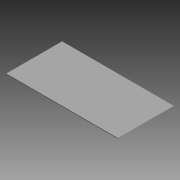
# Autodesk Inventor part: Abtropfgitter
Saved by Autodesk Inventor 2013 (Build 170138000, 138)
## iProperties
Created: 2012-07-26
Part Number: Abtropfgitter
Material: Allgemein
Document SubType Name: Modeling
Designer: fivef
Density: 1 g/cm^3
Mass: 14.3451 g
Surface Area: 368.301 cm^2
Volume: 14.3451 cm^3
Author: fivef
Autodesk Inventor part; units mm, degrees
ref_plane "YZ Plane" through (0, 0, 0) normal (1, 0, 0) x (0, 1, 0)
ref_plane "XZ Plane" through (0, 0, 0) normal (0, 1, 0) x (-1, 0, 0)
ref_plane "XY Plane" through (0, 0, 0) normal (0, 0, 1) x (1, 0, 0)
sketch "Skizze2" plane through (0, 0, 0) normal (0, 0, 1) x (1, 0, 0)
  line L0 (-100, 50) -> (100, 50)
  line L1 (100, 50) -> (100, -50)
  line L2 (100, -50) -> (-100, -50)
  line L3 (-100, -50) -> (-100, 50)
  line L4 (-100, 50) -> (100, -50) construction
  line L5 (100, 50) -> (-100, -50) construction
  circle A0 centre (-98, 48) radius 1.5
  circle A1 centre (-93, 48) radius 1.5
  circle A2 centre (-88, 48) radius 1.5
  circle A3 centre (-83, 48) radius 1.5
  circle A4 centre (-78, 48) radius 1.5
  circle A5 centre (-73, 48) radius 1.5
  circle A6 centre (-68, 48) radius 1.5
  circle A7 centre (-63, 48) radius 1.5
  circle A8 centre (-58, 48) radius 1.5
  circle A9 centre (-53, 48) radius 1.5
  circle A10 centre (-48, 48) radius 1.5
  circle A11 centre (-43, 48) radius 1.5
  circle A12 centre (-38, 48) radius 1.5
  circle A13 centre (-33, 48) radius 1.5
  circle A14 centre (-28, 48) radius 1.5
  circle A15 centre (-23, 48) radius 1.5
  circle A16 centre (-18, 48) radius 1.5
  circle A17 centre (-13, 48) radius 1.5
  circle A18 centre (-8, 48) radius 1.5
  circle A19 centre (-3, 48) radius 1.5
  circle A20 centre (2, 48) radius 1.5
  circle A21 centre (7, 48) radius 1.5
  circle A22 centre (12, 48) radius 1.5
  circle A23 centre (17, 48) radius 1.5
  circle A24 centre (22, 48) radius 1.5
  circle A25 centre (27, 48) radius 1.5
  circle A26 centre (32, 48) radius 1.5
  circle A27 centre (37, 48) radius 1.5
  circle A28 centre (42, 48) radius 1.5
  circle A29 centre (47, 48) radius 1.5
  circle A30 centre (52, 48) radius 1.5
  circle A31 centre (57, 48) radius 1.5
  circle A32 centre (62, 48) radius 1.5
  circle A33 centre (67, 48) radius 1.5
  circle A34 centre (72, 48) radius 1.5
  circle A35 centre (77, 48) radius 1.5
  circle A36 centre (82, 48) radius 1.5
  circle A37 centre (87, 48) radius 1.5
  circle A38 centre (92, 48) radius 1.5
  circle A39 centre (97, 48) radius 1.5
  circle A40 centre (-98, 43) radius 1.5
  circle A41 centre (-93, 43) radius 1.5
  circle A42 centre (-88, 43) radius 1.5
  circle A43 centre (-83, 43) radius 1.5
  circle A44 centre (-78, 43) radius 1.5
  circle A45 centre (-73, 43) radius 1.5
  circle A46 centre (-68, 43) radius 1.5
  circle A47 centre (-63, 43) radius 1.5
  circle A48 centre (-58, 43) radius 1.5
  circle A49 centre (-53, 43) radius 1.5
  circle A50 centre (-48, 43) radius 1.5
  circle A51 centre (-43, 43) radius 1.5
  circle A52 centre (-38, 43) radius 1.5
  circle A53 centre (-33, 43) radius 1.5
  circle A54 centre (-28, 43) radius 1.5
  circle A55 centre (-23, 43) radius 1.5
  circle A56 centre (-18, 43) radius 1.5
  circle A57 centre (-13, 43) radius 1.5
  circle A58 centre (-8, 43) radius 1.5
  circle A59 centre (-3, 43) radius 1.5
  circle A60 centre (2, 43) radius 1.5
  circle A61 centre (7, 43) radius 1.5
  circle A62 centre (12, 43) radius 1.5
  circle A63 centre (17, 43) radius 1.5
  circle A64 centre (22, 43) radius 1.5
  circle A65 centre (27, 43) radius 1.5
  circle A66 centre (32, 43) radius 1.5
  circle A67 centre (37, 43) radius 1.5
  circle A68 centre (42, 43) radius 1.5
  circle A69 centre (47, 43) radius 1.5
  circle A70 centre (52, 43) radius 1.5
  circle A71 centre (57, 43) radius 1.5
  circle A72 centre (62, 43) radius 1.5
  circle A73 centre (67, 43) radius 1.5
  circle A74 centre (72, 43) radius 1.5
  circle A75 centre (77, 43) radius 1.5
  circle A76 centre (82, 43) radius 1.5
  circle A77 centre (87, 43) radius 1.5
  circle A78 centre (92, 43) radius 1.5
  circle A79 centre (97, 43) radius 1.5
  circle A80 centre (-98, 38) radius 1.5
  circle A81 centre (-93, 38) radius 1.5
  circle A82 centre (-88, 38) radius 1.5
  circle A83 centre (-83, 38) radius 1.5
  circle A84 centre (-78, 38) radius 1.5
  circle A85 centre (-73, 38) radius 1.5
  circle A86 centre (-68, 38) radius 1.5
  circle A87 centre (-63, 38) radius 1.5
  circle A88 centre (-58, 38) radius 1.5
  circle A89 centre (-53, 38) radius 1.5
  circle A90 centre (-48, 38) radius 1.5
  circle A91 centre (-43, 38) radius 1.5
  circle A92 centre (-38, 38) radius 1.5
  circle A93 centre (-33, 38) radius 1.5
  circle A94 centre (-28, 38) radius 1.5
  circle A95 centre (-23, 38) radius 1.5
  circle A96 centre (-18, 38) radius 1.5
  circle A97 centre (-13, 38) radius 1.5
  circle A98 centre (-8, 38) radius 1.5
  circle A99 centre (-3, 38) radius 1.5
  circle A100 centre (2, 38) radius 1.5
  circle A101 centre (7, 38) radius 1.5
  circle A102 centre (12, 38) radius 1.5
  circle A103 centre (17, 38) radius 1.5
  circle A104 centre (22, 38) radius 1.5
  circle A105 centre (27, 38) radius 1.5
  circle A106 centre (32, 38) radius 1.5
  circle A107 centre (37, 38) radius 1.5
  circle A108 centre (42, 38) radius 1.5
  circle A109 centre (47, 38) radius 1.5
  circle A110 centre (52, 38) radius 1.5
  circle A111 centre (57, 38) radius 1.5
  circle A112 centre (62, 38) radius 1.5
  circle A113 centre (67, 38) radius 1.5
  circle A114 centre (72, 38) radius 1.5
  circle A115 centre (77, 38) radius 1.5
  circle A116 centre (82, 38) radius 1.5
  circle A117 centre (87, 38) radius 1.5
  circle A118 centre (92, 38) radius 1.5
  circle A119 centre (97, 38) radius 1.5
  circle A120 centre (-98, 33) radius 1.5
  circle A121 centre (-93, 33) radius 1.5
  circle A122 centre (-88, 33) radius 1.5
  circle A123 centre (-83, 33) radius 1.5
  circle A124 centre (-78, 33) radius 1.5
  circle A125 centre (-73, 33) radius 1.5
  circle A126 centre (-68, 33) radius 1.5
  circle A127 centre (-63, 33) radius 1.5
  circle A128 centre (-58, 33) radius 1.5
  circle A129 centre (-53, 33) radius 1.5
  circle A130 centre (-48, 33) radius 1.5
  circle A131 centre (-43, 33) radius 1.5
  circle A132 centre (-38, 33) radius 1.5
  circle A133 centre (-33, 33) radius 1.5
  circle A134 centre (-28, 33) radius 1.5
  circle A135 centre (-23, 33) radius 1.5
  circle A136 centre (-18, 33) radius 1.5
  circle A137 centre (-13, 33) radius 1.5
  circle A138 centre (-8, 33) radius 1.5
  circle A139 centre (-3, 33) radius 1.5
  circle A140 centre (2, 33) radius 1.5
  circle A141 centre (7, 33) radius 1.5
  circle A142 centre (12, 33) radius 1.5
  circle A143 centre (17, 33) radius 1.5
  circle A144 centre (22, 33) radius 1.5
  circle A145 centre (27, 33) radius 1.5
  circle A146 centre (32, 33) radius 1.5
  circle A147 centre (37, 33) radius 1.5
  circle A148 centre (42, 33) radius 1.5
  circle A149 centre (47, 33) radius 1.5
  circle A150 centre (52, 33) radius 1.5
  circle A151 centre (57, 33) radius 1.5
  circle A152 centre (62, 33) radius 1.5
  circle A153 centre (67, 33) radius 1.5
  circle A154 centre (72, 33) radius 1.5
  circle A155 centre (77, 33) radius 1.5
  circle A156 centre (82, 33) radius 1.5
  circle A157 centre (87, 33) radius 1.5
  circle A158 centre (92, 33) radius 1.5
  circle A159 centre (97, 33) radius 1.5
  circle A160 centre (-98, 28) radius 1.5
  circle A161 centre (-93, 28) radius 1.5
  circle A162 centre (-88, 28) radius 1.5
  circle A163 centre (-83, 28) radius 1.5
  circle A164 centre (-78, 28) radius 1.5
  circle A165 centre (-73, 28) radius 1.5
  circle A166 centre (-68, 28) radius 1.5
  circle A167 centre (-63, 28) radius 1.5
  circle A168 centre (-58, 28) radius 1.5
  circle A169 centre (-53, 28) radius 1.5
  circle A170 centre (-48, 28) radius 1.5
  circle A171 centre (-43, 28) radius 1.5
  circle A172 centre (-38, 28) radius 1.5
  circle A173 centre (-33, 28) radius 1.5
  circle A174 centre (-28, 28) radius 1.5
  circle A175 centre (-23, 28) radius 1.5
  circle A176 centre (-18, 28) radius 1.5
  circle A177 centre (-13, 28) radius 1.5
  circle A178 centre (-8, 28) radius 1.5
  circle A179 centre (-3, 28) radius 1.5
  circle A180 centre (2, 28) radius 1.5
  circle A181 centre (7, 28) radius 1.5
  circle A182 centre (12, 28) radius 1.5
  circle A183 centre (17, 28) radius 1.5
  circle A184 centre (22, 28) radius 1.5
  circle A185 centre (27, 28) radius 1.5
  circle A186 centre (32, 28) radius 1.5
  circle A187 centre (37, 28) radius 1.5
  circle A188 centre (42, 28) radius 1.5
  circle A189 centre (47, 28) radius 1.5
  circle A190 centre (52, 28) radius 1.5
  circle A191 centre (57, 28) radius 1.5
  circle A192 centre (62, 28) radius 1.5
  circle A193 centre (67, 28) radius 1.5
  circle A194 centre (72, 28) radius 1.5
  circle A195 centre (77, 28) radius 1.5
  circle A196 centre (82, 28) radius 1.5
  circle A197 centre (87, 28) radius 1.5
  circle A198 centre (92, 28) radius 1.5
  circle A199 centre (97, 28) radius 1.5
  circle A200 centre (-98, 23) radius 1.5
  circle A201 centre (-93, 23) radius 1.5
  circle A202 centre (-88, 23) radius 1.5
  circle A203 centre (-83, 23) radius 1.5
  circle A204 centre (-78, 23) radius 1.5
  circle A205 centre (-73, 23) radius 1.5
  circle A206 centre (-68, 23) radius 1.5
  circle A207 centre (-63, 23) radius 1.5
  circle A208 centre (-58, 23) radius 1.5
  circle A209 centre (-53, 23) radius 1.5
  circle A210 centre (-48, 23) radius 1.5
  circle A211 centre (-43, 23) radius 1.5
  circle A212 centre (-38, 23) radius 1.5
  circle A213 centre (-33, 23) radius 1.5
  circle A214 centre (-28, 23) radius 1.5
  circle A215 centre (-23, 23) radius 1.5
  circle A216 centre (-18, 23) radius 1.5
  circle A217 centre (-13, 23) radius 1.5
  circle A218 centre (-8, 23) radius 1.5
  circle A219 centre (-3, 23) radius 1.5
  circle A220 centre (2, 23) radius 1.5
  circle A221 centre (7, 23) radius 1.5
  circle A222 centre (12, 23) radius 1.5
  circle A223 centre (17, 23) radius 1.5
  circle A224 centre (22, 23) radius 1.5
  circle A225 centre (27, 23) radius 1.5
  circle A226 centre (32, 23) radius 1.5
  circle A227 centre (37, 23) radius 1.5
  circle A228 centre (42, 23) radius 1.5
  circle A229 centre (47, 23) radius 1.5
  circle A230 centre (52, 23) radius 1.5
  circle A231 centre (57, 23) radius 1.5
  circle A232 centre (62, 23) radius 1.5
  circle A233 centre (67, 23) radius 1.5
  circle A234 centre (72, 23) radius 1.5
  circle A235 centre (77, 23) radius 1.5
  circle A236 centre (82, 23) radius 1.5
  circle A237 centre (87, 23) radius 1.5
  circle A238 centre (92, 23) radius 1.5
  circle A239 centre (97, 23) radius 1.5
  circle A240 centre (-98, 18) radius 1.5
  circle A241 centre (-93, 18) radius 1.5
  circle A242 centre (-88, 18) radius 1.5
  circle A243 centre (-83, 18) radius 1.5
  circle A244 centre (-78, 18) radius 1.5
  circle A245 centre (-73, 18) radius 1.5
  circle A246 centre (-68, 18) radius 1.5
  circle A247 centre (-63, 18) radius 1.5
  circle A248 centre (-58, 18) radius 1.5
  circle A249 centre (-53, 18) radius 1.5
  circle A250 centre (-48, 18) radius 1.5
  circle A251 centre (-43, 18) radius 1.5
  circle A252 centre (-38, 18) radius 1.5
  circle A253 centre (-33, 18) radius 1.5
  circle A254 centre (-28, 18) radius 1.5
  circle A255 centre (-23, 18) radius 1.5
  circle A256 centre (-18, 18) radius 1.5
  circle A257 centre (-13, 18) radius 1.5
  circle A258 centre (-8, 18) radius 1.5
  circle A259 centre (-3, 18) radius 1.5
  circle A260 centre (2, 18) radius 1.5
  circle A261 centre (7, 18) radius 1.5
  circle A262 centre (12, 18) radius 1.5
  circle A263 centre (17, 18) radius 1.5
  circle A264 centre (22, 18) radius 1.5
  circle A265 centre (27, 18) radius 1.5
  circle A266 centre (32, 18) radius 1.5
  circle A267 centre (37, 18) radius 1.5
  circle A268 centre (42, 18) radius 1.5
  circle A269 centre (47, 18) radius 1.5
  circle A270 centre (52, 18) radius 1.5
  circle A271 centre (57, 18) radius 1.5
  circle A272 centre (62, 18) radius 1.5
  circle A273 centre (67, 18) radius 1.5
  circle A274 centre (72, 18) radius 1.5
  circle A275 centre (77, 18) radius 1.5
  circle A276 centre (82, 18) radius 1.5
  circle A277 centre (87, 18) radius 1.5
  circle A278 centre (92, 18) radius 1.5
  circle A279 centre (97, 18) radius 1.5
  circle A280 centre (-98, 13) radius 1.5
  circle A281 centre (-93, 13) radius 1.5
  circle A282 centre (-88, 13) radius 1.5
  circle A283 centre (-83, 13) radius 1.5
  circle A284 centre (-78, 13) radius 1.5
  circle A285 centre (-73, 13) radius 1.5
  circle A286 centre (-68, 13) radius 1.5
  circle A287 centre (-63, 13) radius 1.5
  circle A288 centre (-58, 13) radius 1.5
  circle A289 centre (-53, 13) radius 1.5
  circle A290 centre (-48, 13) radius 1.5
  circle A291 centre (-43, 13) radius 1.5
  circle A292 centre (-38, 13) radius 1.5
  circle A293 centre (-33, 13) radius 1.5
  circle A294 centre (-28, 13) radius 1.5
  circle A295 centre (-23, 13) radius 1.5
  circle A296 centre (-18, 13) radius 1.5
  circle A297 centre (-13, 13) radius 1.5
  circle A298 centre (-8, 13) radius 1.5
  circle A299 centre (-3, 13) radius 1.5
  circle A300 centre (2, 13) radius 1.5
  circle A301 centre (7, 13) radius 1.5
  circle A302 centre (12, 13) radius 1.5
  circle A303 centre (17, 13) radius 1.5
  circle A304 centre (22, 13) radius 1.5
  circle A305 centre (27, 13) radius 1.5
  circle A306 centre (32, 13) radius 1.5
  circle A307 centre (37, 13) radius 1.5
  circle A308 centre (42, 13) radius 1.5
  circle A309 centre (47, 13) radius 1.5
  circle A310 centre (52, 13) radius 1.5
  circle A311 centre (57, 13) radius 1.5
  circle A312 centre (62, 13) radius 1.5
  circle A313 centre (67, 13) radius 1.5
  circle A314 centre (72, 13) radius 1.5
  circle A315 centre (77, 13) radius 1.5
  circle A316 centre (82, 13) radius 1.5
  circle A317 centre (87, 13) radius 1.5
  circle A318 centre (92, 13) radius 1.5
  circle A319 centre (97, 13) radius 1.5
  circle A320 centre (-98, 8) radius 1.5
  circle A321 centre (-93, 8) radius 1.5
  circle A322 centre (-88, 8) radius 1.5
  circle A323 centre (-83, 8) radius 1.5
  circle A324 centre (-78, 8) radius 1.5
  circle A325 centre (-73, 8) radius 1.5
  circle A326 centre (-68, 8) radius 1.5
  circle A327 centre (-63, 8) radius 1.5
  circle A328 centre (-58, 8) radius 1.5
  circle A329 centre (-53, 8) radius 1.5
  circle A330 centre (-48, 8) radius 1.5
  circle A331 centre (-43, 8) radius 1.5
  circle A332 centre (-38, 8) radius 1.5
  circle A333 centre (-33, 8) radius 1.5
  circle A334 centre (-28, 8) radius 1.5
  circle A335 centre (-23, 8) radius 1.5
  circle A336 centre (-18, 8) radius 1.5
  circle A337 centre (-13, 8) radius 1.5
  circle A338 centre (-8, 8) radius 1.5
  circle A339 centre (-3, 8) radius 1.5
  circle A340 centre (2, 8) radius 1.5
  circle A341 centre (7, 8) radius 1.5
  circle A342 centre (12, 8) radius 1.5
  circle A343 centre (17, 8) radius 1.5
  circle A344 centre (22, 8) radius 1.5
  circle A345 centre (27, 8) radius 1.5
  circle A346 centre (32, 8) radius 1.5
  circle A347 centre (37, 8) radius 1.5
  circle A348 centre (42, 8) radius 1.5
  circle A349 centre (47, 8) radius 1.5
  circle A350 centre (52, 8) radius 1.5
  circle A351 centre (57, 8) radius 1.5
  circle A352 centre (62, 8) radius 1.5
  circle A353 centre (67, 8) radius 1.5
  circle A354 centre (72, 8) radius 1.5
  circle A355 centre (77, 8) radius 1.5
  circle A356 centre (82, 8) radius 1.5
  circle A357 centre (87, 8) radius 1.5
  circle A358 centre (92, 8) radius 1.5
  circle A359 centre (97, 8) radius 1.5
  circle A360 centre (-98, 3) radius 1.5
  circle A361 centre (-93, 3) radius 1.5
  circle A362 centre (-88, 3) radius 1.5
  circle A363 centre (-83, 3) radius 1.5
  circle A364 centre (-78, 3) radius 1.5
  circle A365 centre (-73, 3) radius 1.5
  circle A366 centre (-68, 3) radius 1.5
  circle A367 centre (-63, 3) radius 1.5
  circle A368 centre (-58, 3) radius 1.5
  circle A369 centre (-53, 3) radius 1.5
  circle A370 centre (-48, 3) radius 1.5
  circle A371 centre (-43, 3) radius 1.5
  circle A372 centre (-38, 3) radius 1.5
  circle A373 centre (-33, 3) radius 1.5
  circle A374 centre (-28, 3) radius 1.5
  circle A375 centre (-23, 3) radius 1.5
  circle A376 centre (-18, 3) radius 1.5
  circle A377 centre (-13, 3) radius 1.5
  circle A378 centre (-8, 3) radius 1.5
  circle A379 centre (-3, 3) radius 1.5
  circle A380 centre (2, 3) radius 1.5
  circle A381 centre (7, 3) radius 1.5
  circle A382 centre (12, 3) radius 1.5
  circle A383 centre (17, 3) radius 1.5
  circle A384 centre (22, 3) radius 1.5
  circle A385 centre (27, 3) radius 1.5
  circle A386 centre (32, 3) radius 1.5
  circle A387 centre (37, 3) radius 1.5
  circle A388 centre (42, 3) radius 1.5
  circle A389 centre (47, 3) radius 1.5
  circle A390 centre (52, 3) radius 1.5
  circle A391 centre (57, 3) radius 1.5
  circle A392 centre (62, 3) radius 1.5
  circle A393 centre (67, 3) radius 1.5
  circle A394 centre (72, 3) radius 1.5
  circle A395 centre (77, 3) radius 1.5
  circle A396 centre (82, 3) radius 1.5
  circle A397 centre (87, 3) radius 1.5
  circle A398 centre (92, 3) radius 1.5
  circle A399 centre (97, 3) radius 1.5
  circle A400 centre (-98, -2) radius 1.5
  circle A401 centre (-93, -2) radius 1.5
  circle A402 centre (-88, -2) radius 1.5
  circle A403 centre (-83, -2) radius 1.5
  circle A404 centre (-78, -2) radius 1.5
  circle A405 centre (-73, -2) radius 1.5
  circle A406 centre (-68, -2) radius 1.5
  circle A407 centre (-63, -2) radius 1.5
  circle A408 centre (-58, -2) radius 1.5
  circle A409 centre (-53, -2) radius 1.5
  circle A410 centre (-48, -2) radius 1.5
  circle A411 centre (-43, -2) radius 1.5
  circle A412 centre (-38, -2) radius 1.5
  circle A413 centre (-33, -2) radius 1.5
  circle A414 centre (-28, -2) radius 1.5
  circle A415 centre (-23, -2) radius 1.5
  circle A416 centre (-18, -2) radius 1.5
  circle A417 centre (-13, -2) radius 1.5
  circle A418 centre (-8, -2) radius 1.5
  circle A419 centre (-3, -2) radius 1.5
  circle A420 centre (2, -2) radius 1.5
  circle A421 centre (7, -2) radius 1.5
  circle A422 centre (12, -2) radius 1.5
  circle A423 centre (17, -2) radius 1.5
  circle A424 centre (22, -2) radius 1.5
  circle A425 centre (27, -2) radius 1.5
  circle A426 centre (32, -2) radius 1.5
  circle A427 centre (37, -2) radius 1.5
  circle A428 centre (42, -2) radius 1.5
  circle A429 centre (47, -2) radius 1.5
  circle A430 centre (52, -2) radius 1.5
  circle A431 centre (57, -2) radius 1.5
  circle A432 centre (62, -2) radius 1.5
  circle A433 centre (67, -2) radius 1.5
  circle A434 centre (72, -2) radius 1.5
  circle A435 centre (77, -2) radius 1.5
  circle A436 centre (82, -2) radius 1.5
  circle A437 centre (87, -2) radius 1.5
  circle A438 centre (92, -2) radius 1.5
  circle A439 centre (97, -2) radius 1.5
  circle A440 centre (-98, -7) radius 1.5
  circle A441 centre (-93, -7) radius 1.5
  circle A442 centre (-88, -7) radius 1.5
  circle A443 centre (-83, -7) radius 1.5
  circle A444 centre (-78, -7) radius 1.5
  circle A445 centre (-73, -7) radius 1.5
  circle A446 centre (-68, -7) radius 1.5
  circle A447 centre (-63, -7) radius 1.5
  circle A448 centre (-58, -7) radius 1.5
  circle A449 centre (-53, -7) radius 1.5
  circle A450 centre (-48, -7) radius 1.5
  circle A451 centre (-43, -7) radius 1.5
  circle A452 centre (-38, -7) radius 1.5
  circle A453 centre (-33, -7) radius 1.5
  circle A454 centre (-28, -7) radius 1.5
  circle A455 centre (-23, -7) radius 1.5
  circle A456 centre (-18, -7) radius 1.5
  circle A457 centre (-13, -7) radius 1.5
  circle A458 centre (-8, -7) radius 1.5
  circle A459 centre (-3, -7) radius 1.5
  circle A460 centre (2, -7) radius 1.5
  circle A461 centre (7, -7) radius 1.5
  circle A462 centre (12, -7) radius 1.5
  circle A463 centre (17, -7) radius 1.5
  circle A464 centre (22, -7) radius 1.5
  circle A465 centre (27, -7) radius 1.5
  circle A466 centre (32, -7) radius 1.5
  circle A467 centre (37, -7) radius 1.5
  circle A468 centre (42, -7) radius 1.5
  circle A469 centre (47, -7) radius 1.5
  circle A470 centre (52, -7) radius 1.5
  circle A471 centre (57, -7) radius 1.5
  circle A472 centre (62, -7) radius 1.5
  circle A473 centre (67, -7) radius 1.5
  circle A474 centre (72, -7) radius 1.5
  circle A475 centre (77, -7) radius 1.5
  circle A476 centre (82, -7) radius 1.5
  circle A477 centre (87, -7) radius 1.5
  circle A478 centre (92, -7) radius 1.5
  circle A479 centre (97, -7) radius 1.5
  circle A480 centre (-98, -12) radius 1.5
  circle A481 centre (-93, -12) radius 1.5
  circle A482 centre (-88, -12) radius 1.5
  circle A483 centre (-83, -12) radius 1.5
  circle A484 centre (-78, -12) radius 1.5
  circle A485 centre (-73, -12) radius 1.5
  circle A486 centre (-68, -12) radius 1.5
  circle A487 centre (-63, -12) radius 1.5
  circle A488 centre (-58, -12) radius 1.5
  circle A489 centre (-53, -12) radius 1.5
  circle A490 centre (-48, -12) radius 1.5
  circle A491 centre (-43, -12) radius 1.5
  circle A492 centre (-38, -12) radius 1.5
  circle A493 centre (-33, -12) radius 1.5
  circle A494 centre (-28, -12) radius 1.5
  circle A495 centre (-23, -12) radius 1.5
  circle A496 centre (-18, -12) radius 1.5
  circle A497 centre (-13, -12) radius 1.5
  circle A498 centre (-8, -12) radius 1.5
  circle A499 centre (-3, -12) radius 1.5
  circle A500 centre (2, -12) radius 1.5
  circle A501 centre (7, -12) radius 1.5
  circle A502 centre (12, -12) radius 1.5
  circle A503 centre (17, -12) radius 1.5
  circle A504 centre (22, -12) radius 1.5
  circle A505 centre (27, -12) radius 1.5
  circle A506 centre (32, -12) radius 1.5
  circle A507 centre (37, -12) radius 1.5
  circle A508 centre (42, -12) radius 1.5
  circle A509 centre (47, -12) radius 1.5
  circle A510 centre (52, -12) radius 1.5
  circle A511 centre (57, -12) radius 1.5
  circle A512 centre (62, -12) radius 1.5
  circle A513 centre (67, -12) radius 1.5
  circle A514 centre (72, -12) radius 1.5
  circle A515 centre (77, -12) radius 1.5
  circle A516 centre (82, -12) radius 1.5
  circle A517 centre (87, -12) radius 1.5
  circle A518 centre (92, -12) radius 1.5
  circle A519 centre (97, -12) radius 1.5
  circle A520 centre (-98, -17) radius 1.5
  circle A521 centre (-93, -17) radius 1.5
  circle A522 centre (-88, -17) radius 1.5
  circle A523 centre (-83, -17) radius 1.5
  circle A524 centre (-78, -17) radius 1.5
  circle A525 centre (-73, -17) radius 1.5
  circle A526 centre (-68, -17) radius 1.5
  circle A527 centre (-63, -17) radius 1.5
  circle A528 centre (-58, -17) radius 1.5
  circle A529 centre (-53, -17) radius 1.5
  circle A530 centre (-48, -17) radius 1.5
  circle A531 centre (-43, -17) radius 1.5
  circle A532 centre (-38, -17) radius 1.5
  circle A533 centre (-33, -17) radius 1.5
  circle A534 centre (-28, -17) radius 1.5
  circle A535 centre (-23, -17) radius 1.5
  circle A536 centre (-18, -17) radius 1.5
  circle A537 centre (-13, -17) radius 1.5
  circle A538 centre (-8, -17) radius 1.5
  circle A539 centre (-3, -17) radius 1.5
  circle A540 centre (2, -17) radius 1.5
  circle A541 centre (7, -17) radius 1.5
  circle A542 centre (12, -17) radius 1.5
  circle A543 centre (17, -17) radius 1.5
  circle A544 centre (22, -17) radius 1.5
  circle A545 centre (27, -17) radius 1.5
  circle A546 centre (32, -17) radius 1.5
  circle A547 centre (37, -17) radius 1.5
  circle A548 centre (42, -17) radius 1.5
  circle A549 centre (47, -17) radius 1.5
  circle A550 centre (52, -17) radius 1.5
  circle A551 centre (57, -17) radius 1.5
  circle A552 centre (62, -17) radius 1.5
  circle A553 centre (67, -17) radius 1.5
  circle A554 centre (72, -17) radius 1.5
  circle A555 centre (77, -17) radius 1.5
  circle A556 centre (82, -17) radius 1.5
  circle A557 centre (87, -17) radius 1.5
  circle A558 centre (92, -17) radius 1.5
  circle A559 centre (97, -17) radius 1.5
  circle A560 centre (-98, -22) radius 1.5
  circle A561 centre (-93, -22) radius 1.5
  circle A562 centre (-88, -22) radius 1.5
  circle A563 centre (-83, -22) radius 1.5
  circle A564 centre (-78, -22) radius 1.5
  circle A565 centre (-73, -22) radius 1.5
  circle A566 centre (-68, -22) radius 1.5
  circle A567 centre (-63, -22) radius 1.5
  circle A568 centre (-58, -22) radius 1.5
  circle A569 centre (-53, -22) radius 1.5
  circle A570 centre (-48, -22) radius 1.5
  circle A571 centre (-43, -22) radius 1.5
  circle A572 centre (-38, -22) radius 1.5
  circle A573 centre (-33, -22) radius 1.5
  circle A574 centre (-28, -22) radius 1.5
  circle A575 centre (-23, -22) radius 1.5
  circle A576 centre (-18, -22) radius 1.5
  circle A577 centre (-13, -22) radius 1.5
  circle A578 centre (-8, -22) radius 1.5
  circle A579 centre (-3, -22) radius 1.5
  circle A580 centre (2, -22) radius 1.5
  circle A581 centre (7, -22) radius 1.5
  circle A582 centre (12, -22) radius 1.5
  circle A583 centre (17, -22) radius 1.5
  circle A584 centre (22, -22) radius 1.5
  circle A585 centre (27, -22) radius 1.5
  circle A586 centre (32, -22) radius 1.5
  circle A587 centre (37, -22) radius 1.5
  circle A588 centre (42, -22) radius 1.5
  circle A589 centre (47, -22) radius 1.5
  circle A590 centre (52, -22) radius 1.5
  circle A591 centre (57, -22) radius 1.5
  circle A592 centre (62, -22) radius 1.5
  circle A593 centre (67, -22) radius 1.5
  circle A594 centre (72, -22) radius 1.5
  circle A595 centre (77, -22) radius 1.5
  circle A596 centre (82, -22) radius 1.5
  circle A597 centre (87, -22) radius 1.5
  circle A598 centre (92, -22) radius 1.5
  circle A599 centre (97, -22) radius 1.5
  circle A600 centre (-98, -27) radius 1.5
  circle A601 centre (-93, -27) radius 1.5
  circle A602 centre (-88, -27) radius 1.5
  circle A603 centre (-83, -27) radius 1.5
  circle A604 centre (-78, -27) radius 1.5
  circle A605 centre (-73, -27) radius 1.5
  circle A606 centre (-68, -27) radius 1.5
  circle A607 centre (-63, -27) radius 1.5
  circle A608 centre (-58, -27) radius 1.5
  circle A609 centre (-53, -27) radius 1.5
  circle A610 centre (-48, -27) radius 1.5
  circle A611 centre (-43, -27) radius 1.5
  circle A612 centre (-38, -27) radius 1.5
  circle A613 centre (-33, -27) radius 1.5
  circle A614 centre (-28, -27) radius 1.5
  circle A615 centre (-23, -27) radius 1.5
  circle A616 centre (-18, -27) radius 1.5
  circle A617 centre (-13, -27) radius 1.5
  circle A618 centre (-8, -27) radius 1.5
  circle A619 centre (-3, -27) radius 1.5
  circle A620 centre (2, -27) radius 1.5
  circle A621 centre (7, -27) radius 1.5
  circle A622 centre (12, -27) radius 1.5
  circle A623 centre (17, -27) radius 1.5
  circle A624 centre (22, -27) radius 1.5
  circle A625 centre (27, -27) radius 1.5
  circle A626 centre (32, -27) radius 1.5
  circle A627 centre (37, -27) radius 1.5
  circle A628 centre (42, -27) radius 1.5
  circle A629 centre (47, -27) radius 1.5
  circle A630 centre (52, -27) radius 1.5
  circle A631 centre (57, -27) radius 1.5
  circle A632 centre (62, -27) radius 1.5
  circle A633 centre (67, -27) radius 1.5
  circle A634 centre (72, -27) radius 1.5
  circle A635 centre (77, -27) radius 1.5
  circle A636 centre (82, -27) radius 1.5
  circle A637 centre (87, -27) radius 1.5
  circle A638 centre (92, -27) radius 1.5
  circle A639 centre (97, -27) radius 1.5
  circle A640 centre (-98, -32) radius 1.5
  circle A641 centre (-93, -32) radius 1.5
  circle A642 centre (-88, -32) radius 1.5
  circle A643 centre (-83, -32) radius 1.5
  circle A644 centre (-78, -32) radius 1.5
  circle A645 centre (-73, -32) radius 1.5
  circle A646 centre (-68, -32) radius 1.5
  circle A647 centre (-63, -32) radius 1.5
  circle A648 centre (-58, -32) radius 1.5
  circle A649 centre (-53, -32) radius 1.5
  circle A650 centre (-48, -32) radius 1.5
  circle A651 centre (-43, -32) radius 1.5
  circle A652 centre (-38, -32) radius 1.5
  circle A653 centre (-33, -32) radius 1.5
  circle A654 centre (-28, -32) radius 1.5
  circle A655 centre (-23, -32) radius 1.5
  circle A656 centre (-18, -32) radius 1.5
  circle A657 centre (-13, -32) radius 1.5
  circle A658 centre (-8, -32) radius 1.5
  circle A659 centre (-3, -32) radius 1.5
  circle A660 centre (2, -32) radius 1.5
  circle A661 centre (7, -32) radius 1.5
  circle A662 centre (12, -32) radius 1.5
  circle A663 centre (17, -32) radius 1.5
  circle A664 centre (22, -32) radius 1.5
  circle A665 centre (27, -32) radius 1.5
  circle A666 centre (32, -32) radius 1.5
  circle A667 centre (37, -32) radius 1.5
  circle A668 centre (42, -32) radius 1.5
  circle A669 centre (47, -32) radius 1.5
  circle A670 centre (52, -32) radius 1.5
  circle A671 centre (57, -32) radius 1.5
  circle A672 centre (62, -32) radius 1.5
  circle A673 centre (67, -32) radius 1.5
  circle A674 centre (72, -32) radius 1.5
  circle A675 centre (77, -32) radius 1.5
  circle A676 centre (82, -32) radius 1.5
  circle A677 centre (87, -32) radius 1.5
  circle A678 centre (92, -32) radius 1.5
  circle A679 centre (97, -32) radius 1.5
  circle A680 centre (-98, -37) radius 1.5
  circle A681 centre (-93, -37) radius 1.5
  circle A682 centre (-88, -37) radius 1.5
  circle A683 centre (-83, -37) radius 1.5
  circle A684 centre (-78, -37) radius 1.5
  circle A685 centre (-73, -37) radius 1.5
  circle A686 centre (-68, -37) radius 1.5
  circle A687 centre (-63, -37) radius 1.5
  circle A688 centre (-58, -37) radius 1.5
  circle A689 centre (-53, -37) radius 1.5
  circle A690 centre (-48, -37) radius 1.5
  circle A691 centre (-43, -37) radius 1.5
  circle A692 centre (-38, -37) radius 1.5
  circle A693 centre (-33, -37) radius 1.5
  circle A694 centre (-28, -37) radius 1.5
  circle A695 centre (-23, -37) radius 1.5
  circle A696 centre (-18, -37) radius 1.5
  circle A697 centre (-13, -37) radius 1.5
  circle A698 centre (-8, -37) radius 1.5
  circle A699 centre (-3, -37) radius 1.5
  circle A700 centre (2, -37) radius 1.5
  circle A701 centre (7, -37) radius 1.5
  circle A702 centre (12, -37) radius 1.5
  circle A703 centre (17, -37) radius 1.5
  circle A704 centre (22, -37) radius 1.5
  circle A705 centre (27, -37) radius 1.5
  circle A706 centre (32, -37) radius 1.5
  circle A707 centre (37, -37) radius 1.5
  circle A708 centre (42, -37) radius 1.5
  circle A709 centre (47, -37) radius 1.5
  circle A710 centre (52, -37) radius 1.5
  circle A711 centre (57, -37) radius 1.5
  circle A712 centre (62, -37) radius 1.5
  circle A713 centre (67, -37) radius 1.5
  circle A714 centre (72, -37) radius 1.5
  circle A715 centre (77, -37) radius 1.5
  circle A716 centre (82, -37) radius 1.5
  circle A717 centre (87, -37) radius 1.5
  circle A718 centre (92, -37) radius 1.5
  circle A719 centre (97, -37) radius 1.5
  circle A720 centre (-98, -42) radius 1.5
  circle A721 centre (-93, -42) radius 1.5
  circle A722 centre (-88, -42) radius 1.5
  circle A723 centre (-83, -42) radius 1.5
  circle A724 centre (-78, -42) radius 1.5
  circle A725 centre (-73, -42) radius 1.5
  circle A726 centre (-68, -42) radius 1.5
  circle A727 centre (-63, -42) radius 1.5
  circle A728 centre (-58, -42) radius 1.5
  circle A729 centre (-53, -42) radius 1.5
  circle A730 centre (-48, -42) radius 1.5
  circle A731 centre (-43, -42) radius 1.5
  circle A732 centre (-38, -42) radius 1.5
  circle A733 centre (-33, -42) radius 1.5
  circle A734 centre (-28, -42) radius 1.5
  circle A735 centre (-23, -42) radius 1.5
  circle A736 centre (-18, -42) radius 1.5
  circle A737 centre (-13, -42) radius 1.5
  circle A738 centre (-8, -42) radius 1.5
  circle A739 centre (-3, -42) radius 1.5
  circle A740 centre (2, -42) radius 1.5
  circle A741 centre (7, -42) radius 1.5
  circle A742 centre (12, -42) radius 1.5
  circle A743 centre (17, -42) radius 1.5
  circle A744 centre (22, -42) radius 1.5
  circle A745 centre (27, -42) radius 1.5
  circle A746 centre (32, -42) radius 1.5
  circle A747 centre (37, -42) radius 1.5
  circle A748 centre (42, -42) radius 1.5
  circle A749 centre (47, -42) radius 1.5
  circle A750 centre (52, -42) radius 1.5
  circle A751 centre (57, -42) radius 1.5
  circle A752 centre (62, -42) radius 1.5
  circle A753 centre (67, -42) radius 1.5
  circle A754 centre (72, -42) radius 1.5
  circle A755 centre (77, -42) radius 1.5
  circle A756 centre (82, -42) radius 1.5
  circle A757 centre (87, -42) radius 1.5
  circle A758 centre (92, -42) radius 1.5
  circle A759 centre (97, -42) radius 1.5
  circle A760 centre (-98, -47) radius 1.5
  circle A761 centre (-93, -47) radius 1.5
  circle A762 centre (-88, -47) radius 1.5
  circle A763 centre (-83, -47) radius 1.5
  circle A764 centre (-78, -47) radius 1.5
  circle A765 centre (-73, -47) radius 1.5
  circle A766 centre (-68, -47) radius 1.5
  circle A767 centre (-63, -47) radius 1.5
  circle A768 centre (-58, -47) radius 1.5
  circle A769 centre (-53, -47) radius 1.5
  circle A770 centre (-48, -47) radius 1.5
  circle A771 centre (-43, -47) radius 1.5
  circle A772 centre (-38, -47) radius 1.5
  circle A773 centre (-33, -47) radius 1.5
  circle A774 centre (-28, -47) radius 1.5
  circle A775 centre (-23, -47) radius 1.5
  circle A776 centre (-18, -47) radius 1.5
  circle A777 centre (-13, -47) radius 1.5
  circle A778 centre (-8, -47) radius 1.5
  circle A779 centre (-3, -47) radius 1.5
  circle A780 centre (2, -47) radius 1.5
  circle A781 centre (7, -47) radius 1.5
  circle A782 centre (12, -47) radius 1.5
  circle A783 centre (17, -47) radius 1.5
  circle A784 centre (22, -47) radius 1.5
  circle A785 centre (27, -47) radius 1.5
  circle A786 centre (32, -47) radius 1.5
  circle A787 centre (37, -47) radius 1.5
  circle A788 centre (42, -47) radius 1.5
  circle A789 centre (47, -47) radius 1.5
  circle A790 centre (52, -47) radius 1.5
  circle A791 centre (57, -47) radius 1.5
  circle A792 centre (62, -47) radius 1.5
  circle A793 centre (67, -47) radius 1.5
  circle A794 centre (72, -47) radius 1.5
  circle A795 centre (77, -47) radius 1.5
  circle A796 centre (82, -47) radius 1.5
  circle A797 centre (87, -47) radius 1.5
  circle A798 centre (92, -47) radius 1.5
  circle A799 centre (97, -47) radius 1.5
  point P0 (0, 0)
  dimension "d2" = 100
  dimension "d4" = 200
  dimension "d5" = 3
  dimension "d6" = 2
  dimension "d7" = 2
  dimension "d10" = 5
  dimension "d13" = 5
  constraints: 800 centre point, 12 end point, 2 horizontal, 2 midpoint, 2 parallel, 1 perpendicular, 1 vertical, 1598 other
  measures "d2" distance of L2.end L0.start
  measures "d4" distance of L0.start L0.end
  measures "d5" diameter of A0
  measures "d6" distance from line of L0 A0.centre
  measures "d7" distance from line of L3 A0.centre
  measures "d10" distance of A0.centre A1.centre
  measures "d13" distance of A0.centre A40.centre
extrude "Extrusion2" add sketch "Skizze2" along normal blind 1
